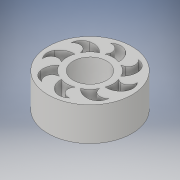
# Autodesk Inventor part: whee
Saved by Autodesk Inventor 2018 (Build 220112000, 112)
## iProperties
Created: 2020-01-09
Part Number: whee
Material: Generic
Document SubType Name: Modeling
Designer: AOFUser
Density: 1 g/cm^3
Appearance: Default
Author: AOFUser
Autodesk Inventor part; units mm, degrees
ref_plane "YZ Plane" through (0, 0, 0) normal (1, 0, 0) x (0, 1, 0)
ref_plane "XZ Plane" through (0, 0, 0) normal (0, 1, 0) x (-1, 0, 0)
ref_plane "XY Plane" through (0, 0, 0) normal (0, 0, 1) x (1, 0, 0)
sketch "Sketch1" plane through (0, 0, 0) normal (0, 1, 0) x (-1, 0, 0)
  circle A0 centre (0, 0) radius 12.7
  circle A1 centre (0, 0) radius 31.75
  dimension "d0" = 25.4
  dimension "d1" = 63.5
  constraints: 2 centre point, 2 coincident
  measures "d0" diameter of A0
  measures "d1" diameter of A1
extrude "Extrusion1" add sketch "Sketch1" along normal blind 25.4
sketch "Sketch2" plane through (0, 25.4, 0) normal (0, 1, 0) x (1, 0, 0)
  circle A0 centre (0, 0) radius 31.75 projected
  line L0 (-31.75, 0) -> (-26.67, 0)
  line L1 (-26.67, 0) -> (-16.51, 0)
  line L2 (-16.51, 5.08) -> (-26.67, 0)
  line L3 (-16.51, -5.08) -> (-26.67, 0)
  arc A1 (-16.51, 5.08) -> (-26.67, 0) centre (-17.3323, -5.9755) ccw
  line L4 (-26.67, 0) -> (-25.783, -10.1212)
  arc A2 (-26.67, 0) -> (-25.783, -10.1212) centre (-19.661, -4.4852) ccw
  arc A3 (-16.51, 5.08) -> (-16.51, -5.08) centre (-4.0157, 0) ccw
  arc A4 (-16.51, -5.08) -> (-25.783, -10.1212) centre (-20.2123, -9.3191) ccw
  dimension "d4" = 5.08
  dimension "d6" = 5.08
  dimension "d7" = 10.16
  dimension "d13" = 10.16
  constraints: 10 end point, 8 point on circle, 4 centre point, 1 horizontal, 1 horizontal alignment, 1 point on line, 1 tangent, 1 other
  measures "d4" distance of L0.start L0.end
  measures "d6" distance of L1.end L3.start
  measures "d7" distance of L3.start L2.start
  measures "d13" distance of L0.end L4.end
extrude "Extrusion2" cut sketch "Sketch2" against normal blind 25.4 contours A1 L2 | L2 A3 L1 | L1 A3 A4 L3 | L3 A4 L4 | L4 A4 A2 | A4 L3 | L4 A4
pattern_circular "Circular Pattern1" count 8 over 360 about axis through (0, 0, 0) along (0, 1, 0) of "Extrusion2"
body "Solid1"
